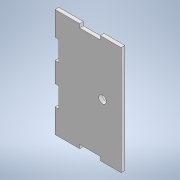
# Autodesk Inventor part: top switch
Saved by Autodesk Inventor 2020 (Build 240168000, 168)
## iProperties
Created: 2022-02-16
Part Number: top switch
Material: Generic
Document SubType Name: Modeling
Designer: rwte
Density: 1 g/cm^3
Appearance: Default
Author: rwte
Autodesk Inventor part; units mm, degrees
ref_plane "YZ Plane" through (0, 0, 0) normal (1, 0, 0) x (0, 1, 0)
ref_plane "XZ Plane" through (0, 0, 0) normal (0, 1, 0) x (-1, 0, 0)
ref_plane "XY Plane" through (0, 0, 0) normal (0, 0, 1) x (1, 0, 0)
sketch "Sketch1" plane through (0, 0, 0) normal (0, 0, 1) x (1, 0, 0)
  line L0 (-30, -40.5) -> (-30, 40.5)
  line L1 (-30, 40.5) -> (30, 40.5)
  line L2 (30, 40.5) -> (30, -40.5)
  line L3 (30, -40.5) -> (-30, -40.5)
  line L4 (-30, -40.5) -> (30, 40.5) construction
  line L5 (-30, 40.5) -> (30, -40.5) construction
  line L6 (-30, 40.5) -> (-10, 40.5)
  line L7 (-10, 40.5) -> (-10, 43.5)
  line L8 (-10, 43.5) -> (-30, 43.5)
  line L9 (-30, 43.5) -> (-30, 40.5) construction
  line L10 (30, 40.5) -> (10, 40.5)
  line L11 (10, 40.5) -> (10, 43.5)
  line L12 (10, 43.5) -> (30, 43.5)
  line L13 (30, 43.5) -> (30, 40.5)
  line L14 (-45.6, 0) -> (42.6, 0) projected
  line L15 (0, -60.9) -> (0, 60.9) projected
  line L16 (-10, -40.5) -> (-10, -43.5)
  line L17 (-10, -43.5) -> (-30, -43.5)
  line L18 (-30, -43.5) -> (-30, -40.5) construction
  line L19 (10, -40.5) -> (10, -43.5)
  line L20 (10, -43.5) -> (30, -43.5)
  line L21 (30, -43.5) -> (30, -40.5)
  line L22 (-30, -40.5) -> (-30, -24.3)
  line L23 (-30, -24.3) -> (-33, -24.3)
  line L24 (-33, -24.3) -> (-33, -40.5)
  line L25 (-33, -40.5) -> (-30, -40.5) construction
  line L26 (-30, -8.1) -> (-30, 8.1)
  line L27 (-30, 8.1) -> (-33, 8.1)
  line L28 (-33, 8.1) -> (-33, -8.1)
  line L29 (-33, -8.1) -> (-30, -8.1)
  line L30 (-30, 40.5) -> (-30, 24.3)
  line L31 (-30, 24.3) -> (-33, 24.3)
  line L32 (-33, 24.3) -> (-33, 40.5)
  line L33 (-33, 40.5) -> (-30, 40.5) construction
  line L34 (-30, 43.5) -> (-33, 43.5)
  line L35 (-33, 43.5) -> (-33, 40.5)
  line L36 (-30, -43.5) -> (-33, -43.5)
  line L37 (-33, -43.5) -> (-33, -40.5)
  point P0 (0, 0)
  point P1 (20, 43.5)
  point P2 (-20, 43.5)
  point P3 (20, -43.5)
  point P4 (-20, -43.5)
  point P5 (-33, 32.4)
  point P6 (-33, 0)
  point P7 (-33, -32.4)
  point P8 (-30, 0)
  dimension "d0" = 81
  dimension "d1" = 60
  dimension "d4" = 20
  dimension "d5" = 20
  dimension "d6" = 3
  dimension "d7" = 3
  dimension "d8" = 16.2
  constraints: 72 end point, 12 parallel, 9 perpendicular, 8 midpoint, 8 symmetric about line, 7 point on line, 2 collinear, 2 horizontal alignment, 2 vertical alignment, 1 horizontal, 1 vertical
  measures "d0" distance of L1.end L2.end
  measures "d1" distance of L0.end L1.end
  measures "d4" distance of L8.end L7.end
  measures "d5" distance of L12.end L11.end
  measures "d6" distance of L1.end L12.end
  measures "d7" distance of L32.end L0.end
  measures "d8" distance of L31.end L32.end
extrude "Extrusion1" add sketch "Sketch1" along normal blind 3
sketch "Sketch2" plane through (0, 0, 3) normal (0, 0, 1) x (1, 0, 0)
  line L0 (-45.6, 0) -> (42.6, 0) projected
  line L1 (0, -60.9) -> (0, 60.9) projected
  circle A0 centre (15, 0) radius 3.05
  line L2 (30, -43.5) -> (30, 43.5) projected
  dimension "d9" = 6.1
  dimension "d12" = 15
  constraints: 1 centre point, 1 coincident, 1 point on line, 1 other
  measures "d9" diameter of A0
  measures "d12" distance from line of L2 point (15, 0)
extrude "Extrusion2" cut sketch "Sketch2" against normal through all
equation "\"d4\" = 0.333333 * d1"
equation "\"d5\" = d4"
equation "\"d6\" = d2"
equation "\"d7\" = d2"
equation "\"d8\" = 0.2 * d0"
equation "\"d2\" = 3"
body "Solid1"
